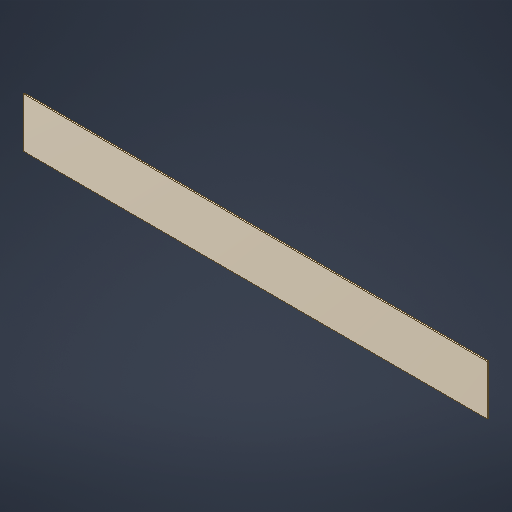
# Autodesk Inventor part: TETHLON_TAPE
Saved by Autodesk Inventor 2026.2 (Build 302298010, 298A)
## iProperties
Created: 2026-04-02
Part Number: TETHLON_TAPE
Material: Iglidur,V400
Document SubType Name: Modeling
Designer: 4aida
Density: 1.49472 g/cm^3
Appearance: Smooth - Light Beige
Author: 4aida
Autodesk Inventor part; units mm, degrees
ref_plane "YZ Plane" through (0, 0, 0) normal (1, 0, 0) x (0, 1, 0)
ref_plane "XZ Plane" through (0, 0, 0) normal (0, 1, 0) x (-1, 0, 0)
ref_plane "XY Plane" through (0, 0, 0) normal (0, 0, 1) x (1, 0, 0)
sketch "Sketch1" plane through (0, 0, 0) normal (0, 0, 1) x (1, 0, 0)
  line L0 (88.9, -9.525) -> (-88.9, -9.525)
  line L1 (-88.9, -9.525) -> (-88.9, 9.525)
  line L2 (-88.9, 9.525) -> (88.9, 9.525)
  line L3 (88.9, 9.525) -> (88.9, -9.525)
  line L4 (88.9, -9.525) -> (-88.9, 9.525) construction
  line L5 (-88.9, -9.525) -> (88.9, 9.525) construction
  point P0 (0, 0)
  dimension "d0" = 19.05
  dimension "d1" = 177.8
  constraints: 12 end point, 2 midpoint, 2 parallel, 1 horizontal, 1 perpendicular
  measures "d0" distance of L0.end L1.end
  measures "d1" distance of L1.end L2.end
extrude "Extrusion1" add sketch "Sketch1" along normal blind 0.508
body "Solid1"
